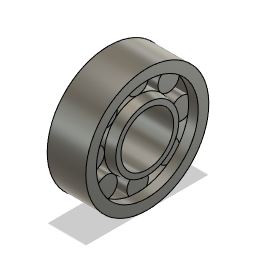
Bearing_GOST_8328-75_42000 v3 (Autodesk Fusion 360 design; units mm, degrees)
Autodesk Fusion 360 part; units mm, degrees
sketch "Sketch1" plane through (0, 0, 0) normal (0, 0, 1) x (1, 0, 0)
  line L0 (-56.5, 0) -> (48.5, 0)
  line L1 (-5.5, 7.5) -> (-5.5, 10.5)
  line L2 (-5.5, 10.5) -> (-2.75, 10.5)
  line L3 (-2.75, 10.5) -> (-2.75, 9.45)
  line L4 (-2.75, 9.45) -> (2.75, 9.45)
  line L5 (2.75, 9.45) -> (5.5, 8.9651)
  line L6 (5.5, 8.9651) -> (5.5, 7.5)
  line L7 (5.5, 7.5) -> (-5.5, 7.5)
  line L8 (-5.5, 14.5) -> (-2.75, 14.5)
  line L9 (-2.75, 14.5) -> (-2.75, 15.55)
  line L10 (-2.75, 15.55) -> (2.75, 15.55)
  line L11 (2.75, 15.55) -> (2.75, 14.5)
  line L12 (2.75, 14.5) -> (5.5, 14.5)
  line L13 (5.5, 14.5) -> (5.5, 17.5)
  line L14 (5.5, 17.5) -> (-5.5, 17.5)
  line L15 (-5.5, 17.5) -> (-5.5, 14.5)
  line L16 (-2.75, 14.5) -> (-2.75, 10.5)
  line L17 (2.75, 14.5) -> (2.75, 9.45)
  line L18 (0, 15.55) -> (0, 9.45) construction
  line L19 (-2.75, 12.5) -> (2.75, 12.5)
  point P0 (0, 7.5)
  point P1 (0, 9.45)
  point P2 (0, 12.5)
  dimension "d1" = 15
  dimension "d2" = 10
  dimension "d3" = 11
  dimension "d4" = 2.75
  dimension "d6" = 35
  dimension "d7" = 31.1
  dimension "d9" = 29
  dimension "d10" = 21
  dimension "d11" = 25
  constraint horizontal L0
  constraint coincident L0 origin
  constraint vertical L1
  constraint perpendicular L1 L2
  constraint perpendicular L2 L3
  constraint perpendicular L1 L4
  constraint perpendicular L4 L6
  constraint perpendicular L6 L7
  constraint coincident L1.start L7.end
  constraint midpoint L7 P0
  constraint vertical origin P0
  constraint midpoint L4 P1
  constraint vertical P0 P1
  constraint horizontal L8
  constraint perpendicular L8 L9
  constraint perpendicular L9 L10
  constraint perpendicular L10 L11
  constraint perpendicular L11 L12
  constraint perpendicular L12 L13
  constraint perpendicular L11 L14
  constraint perpendicular L14 L15
  constraint vertical L2.end L8.end
  constraint vertical L1.end L8.start
  constraint vertical L4.end L11.end
  constraint vertical L5.end L12.end
  constraint horizontal L8.end L11.end
  constraint parallel L11 L17
  constraint midpoint L10 L18.start
  constraint coincident P1 L18.end
  constraint coincident L16 L19.start
  constraint coincident L17 L19.end
  constraint perpendicular L17 L19
  constraint midpoint L18 P2
  constraint coincident L19 P2
  measures "d2" angle of L4 L5
  measures "d3" distance of L1 L6
  measures "d4" horizontal distance of L4.end L5.end
revolve "Revolve1" add sketch "Sketch1" angle 360 about axis through (-56.5, 0, 0) along (1, 0, 0) contours L1 L2 L3 L4 L5 L6 L7 | L8 L9 L10 L11 L12 L13 L14 L15 makes body 1 at (-1.8333, 17.413, -1.7424) makes body 2 at (-1.8333, 7.4627, -0.7468)
revolve "Revolve2" add sketch "Sketch1" angle 360 about axis through (-2.75, 12.5, 0) along (1, 0, 0) separate body contours L9 L10 L11 L16 L17 L19 makes body 3
pattern_circular "C-Pattern1" count 8 over 360 about axis through (-56.5, 0, 0) along (1, 0, 0) of bodies 3 makes body 4 at (-0.9167, 11.1003, 10.8853) makes body 5 at (-0.9167, 0.152, 15.5462) makes body 6 at (-0.9167, -10.8853, 11.1003) makes body 7 at (-0.9167, -15.5462, 0.152) makes body 8 at (-0.9167, -11.1003, -10.8853) makes body 9 at (-0.9167, -0.152, -15.5462) makes body 10 at (-0.9167, 10.8853, -11.1003)
